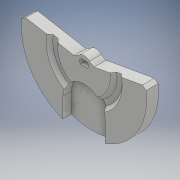
# Autodesk Inventor part: RescueKitThrow-Joint
Saved by Autodesk Inventor 2018.3 (Build 223284000, 284)
## iProperties
Created: 2019-02-13
Part Number: RescueKitThrow-Joint
Material: 一般
Document SubType Name: Modeling
Designer: TOMOKI
Density: 1 g/cm^3
Appearance: 既定
Author: TOMOKI
Autodesk Inventor part; units mm, degrees
ref_plane "YZ Plane" through (0, 0, 0) normal (1, 0, 0) x (0, 1, 0)
ref_plane "XZ Plane" through (0, 0, 0) normal (0, 1, 0) x (-1, 0, 0)
ref_plane "XY Plane" through (0, 0, 0) normal (0, 0, 1) x (1, 0, 0)
sketch "スケッチ1" plane through (0, 0, 0) normal (0, 1, 0) x (-1, 0, 0)
  arc A0 (54.8142, 37.6946) -> (46.9358, 37.6946) centre (50.875, 37) ccw
  circle A1 centre (50.875, 13.875) radius 12.5
  arc A2 (14.4371, 43.425) -> (87.3129, 43.425) centre (50.875, 37) ccw
  line L0 (50.875, 37) -> (87.3129, 43.425)
  line L1 (50.875, 37) -> (87.875, 37) construction
  line L2 (87.3129, 43.425) -> (50.875, 37)
  line L3 (50.875, 37) -> (14.4371, 43.425)
  point P0 (0, 0)
  dimension "d22" = 25
  dimension "d26" = 74
  dimension "d27" = 10
  dimension "d38" = 4
  constraints: 8 end point, 4 point on circle, 3 centre point, 2 point on line, 1 coincident, 1 collinear, 1 equal length, 1 horizontal
  measures "d22" diameter of A1
  measures "d26" diameter of A2
  measures "d27" angle of L1 L0
  measures "d38" radius of A0
extrude "押し出し1" add sketch "スケッチ1" along normal blind 7
sketch "スケッチ2" plane through (0, 7, 0) normal (0, 1, 0) x (1, 0, 0)
  circle A0 centre (-50.875, -13.875) radius 12.5
  circle A1 centre (-50.875, -13.875) radius 12.5
  point P0 (0, 0)
  constraints: 2 centre point, 2 coincident, 1 concentric
extrude "押し出し2" add sketch "スケッチ2" against normal blind 2
sketch "スケッチ3" plane through (0, 0, 0) normal (0, -1, 0) x (1, 0, 0)
  circle A0 centre (-50.875, 13.875) radius 12.5 projected
  arc A1 (-46.9358, 37.6946) -> (-54.8142, 37.6946) centre (-50.875, 37) ccw projected
  circle A2 centre (-50.875, 13.875) radius 12.5 projected
  line L0 (-63.375, 13.875) -> (-38.375, 13.875)
  line L1 (-38.375, 13.875) -> (-38.375, 0)
  line L2 (-38.375, 0) -> (-63.375, 0)
  line L3 (-63.375, 0) -> (-63.375, 13.875)
  line L4 (-54.8142, 37.6946) -> (-87.3129, 43.425) projected
  arc A3 (-87.3129, 43.425) -> (-14.4371, 43.425) centre (-50.875, 37) ccw projected
  line L5 (-14.4371, 43.425) -> (-46.9358, 37.6946) projected
  point P0 (0, 0)
  constraints: 8 end point, 2 parallel, 1 horizontal, 1 horizontal alignment, 1 perpendicular, 1 other
extrude "押し出し3" cut sketch "スケッチ3" against normal blind 5 contours L1 A3 L3 A0 | A0 L0 | L1 L2 A3 | A3 L2 L3 picked at (-53.2419, 10.4459)
sketch "スケッチ4" plane through (0, 0, 0) normal (0, -1, 0) x (1, 0, 0)
  arc A0 (-46.9358, 37.6946) -> (-54.8142, 37.6946) centre (-50.875, 37) ccw projected
  circle A1 centre (-50.875, 37) radius 2.6
  arc A2 (-38.375, 13.875) -> (-63.375, 13.875) centre (-50.875, 13.875) ccw projected
  line L0 (-63.375, 2.1754) -> (-63.375, 13.875) projected
  line L1 (-38.375, 13.875) -> (-38.375, 2.1754) projected
  arc A3 (-38.375, 2.1754) -> (-14.4371, 43.425) centre (-50.875, 37) ccw projected
  line L2 (-14.4371, 43.425) -> (-46.9358, 37.6946) projected
  line L3 (-54.8142, 37.6946) -> (-87.3129, 43.425) projected
  arc A4 (-87.3129, 43.425) -> (-63.375, 2.1754) centre (-50.875, 37) ccw projected
  line L4 (-52.9987, 38.5) -> (-48.7513, 38.5)
  line L5 (-42.875, 38.5) -> (-42.875, 38.4106)
  line L6 (-48.7513, 35.5) -> (-52.9987, 35.5)
  line L7 (-58.875, 38.4106) -> (-58.875, 38.5)
  point P0 (0, 0)
  dimension "d12" = 5.2
  dimension "d47" = 3
  dimension "d48" = 1.5
  constraints: 8 end point, 4 point on circle, 2 parallel, 2 point on line, 1 centre point, 1 coincident, 1 horizontal, 1 perpendicular
  measures "d12" diameter of A1
  measures "d47" distance between parallel lines of L6 L4
  measures "d48" distance from line of A0.centre L4
extrude "押し出し4" cut sketch "スケッチ4" against normal blind 8 contours A1 L6 L4
chamfer "面取り1" distance 2 angle 45 4 edges at (-46.9358, 3.5, 37.6946) (-54.8142, 3.5, 37.6946) (-87.3129, 3.5, 43.425) (-14.4371, 3.5, 43.425)
sketch "スケッチ8" plane through (0, 7, 0) normal (0, 1, 0) x (1, 0, 0)
  line L0 (-14.1432, -41.4467) -> (-16.4067, -43.0777) projected
  arc A0 (-14.1432, -41.4467) -> (-87.6068, -41.4467) centre (-50.875, -37) ccw projected
  line L1 (-85.3433, -43.0777) -> (-87.6068, -41.4467) projected
  line L2 (-85.3433, -43.0777) -> (-56.7838, -38.0419) projected
  line L3 (-53.9856, -39.5148) -> (-56.7838, -38.0419) projected
  arc A1 (-53.9856, -39.5148) -> (-47.7644, -39.5148) centre (-50.875, -37) ccw projected
  line L4 (-44.9662, -38.0419) -> (-47.7644, -39.5148) projected
  line L5 (-44.9662, -38.0419) -> (-16.4067, -43.0777) projected
  point P0 (0, 0)
extrude "押し出し8" [suppressed]
sketch "スケッチ9" plane through (0, 0, 0) normal (0, -1, 0) x (1, 0, 0)
  line L0 (-48.7513, 35.5) -> (-52.9987, 35.5) projected
  arc A0 (-52.9987, 38.5) -> (-52.9987, 35.5) centre (-50.875, 37) ccw projected
  line L1 (-52.9987, 38.5) -> (-48.7513, 38.5) projected
  arc A1 (-48.7513, 35.5) -> (-48.7513, 38.5) centre (-50.875, 37) ccw projected
  line L2 (-16.4067, 43.0777) -> (-14.1432, 41.4467) projected
  line L3 (-16.4067, 43.0777) -> (-44.9662, 38.0419) projected
  line L4 (-47.7644, 39.5148) -> (-44.9662, 38.0419) projected
  arc A2 (-47.7644, 39.5148) -> (-53.9856, 39.5148) centre (-50.875, 37) ccw projected
  line L5 (-56.7838, 38.0419) -> (-53.9856, 39.5148) projected
  line L6 (-56.7838, 38.0419) -> (-85.3433, 43.0777) projected
  line L7 (-87.6068, 41.4467) -> (-85.3433, 43.0777) projected
  arc A3 (-87.6068, 41.4467) -> (-63.375, 2.1754) centre (-50.875, 37) ccw projected
  line L8 (-63.375, 2.1754) -> (-63.375, 13.875) projected
  arc A4 (-38.375, 13.875) -> (-63.375, 13.875) centre (-50.875, 13.875) ccw projected
  line L9 (-38.375, 13.875) -> (-38.375, 2.1754) projected
  arc A5 (-38.375, 2.1754) -> (-14.1432, 41.4467) centre (-50.875, 37) ccw projected
  circle A6 centre (-50.875, 37) radius 17.5
  circle A7 centre (-50.875, 37) radius 20.5
  circle A8 centre (-50.875, 37) radius 19
  point P0 (0, 0)
  dimension "d39" = 35
  dimension "d40" = 41
  dimension "d41" = 38
  constraints: 3 centre point, 3 coincident
  measures "d39" diameter of A6
  measures "d40" diameter of A7
  measures "d41" diameter of A8
extrude "押し出し9" cut sketch "スケッチ9" against normal blind 2 contours L0 A0 L1 A1 | A7 A4 A8 L3 | L3 A8 L6 A7 | A8 A4 A6 L3 | L3 A6 L6 A8 | L6 A8 A4 A7 | L6 A6 A4 A8 | A7 A4 A8 | A8 A4 A6
chamfer "面取り2" distance 2 angle 45 4 edges at (-69.646, 0, 28.7598) (-32.104, 0, 28.7598) (-66.8754, 0, 29.9123) (-34.8746, 0, 29.9123)
